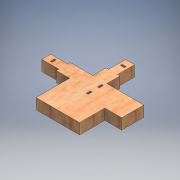
# Autodesk Inventor part: BearingStand_V2
Saved by Autodesk Inventor 2016 (Build 200138000, 138)
## iProperties
Created: 2015-11-23
Part Number: BearingStand_V2
Material: Wood (Birch)
Document SubType Name: Modeling
Designer: m2memari
Density: 0.55 g/cm^3
Appearance: Birch - Natural Polished
BearingDiameter: 24.000 mm
WoodThickness: 6.390 mm
BearingWidth: 7.000 mm
BearingShaftDiameter: 8.000 mm
ZipTieWidth: 2.500 mm
ZipTieThickness: 1.100 mm
ZipTieClearance: 1.000 mm
ZipTieDistance: 10.000 mm
BearingHolderHeight: 24.526 mm
BearingSiliconeWidth: 14.000 mm
Author: m2memari
Autodesk Inventor part; units mm, degrees
ref_plane "YZ Plane" through (0, 0, 0) normal (1, 0, 0) x (0, 1, 0)
ref_plane "XZ Plane" through (0, 0, 0) normal (0, 1, 0) x (-1, 0, 0)
ref_plane "XY Plane" through (0, 0, 0) normal (0, 0, 1) x (1, 0, 0)
sketch "Sketch1" plane through (0, 0, 0) normal (0, 0, 1) x (1, 0, 0)
  line L0 (-2.6473, 22.1) -> (2.6473, 22.1)
  line L1 (2.6473, 22.1) -> (2.6473, 12)
  line L2 (2.6473, 12) -> (4.1473, 12)
  line L3 (4.1473, 12) -> (4.1473, 4.1473)
  line L4 (0, 22.1) -> (0, 0) construction
  line L5 (-2.6473, 22.1) -> (-2.6473, 12)
  line L6 (-2.6473, 12) -> (-4.1473, 12)
  line L7 (-1.25, 18.6) -> (1.25, 18.6)
  line L8 (1.25, 18.6) -> (1.25, 17.5)
  line L9 (1.25, 17.5) -> (-1.25, 17.5)
  line L10 (-1.25, 17.5) -> (-1.25, 18.6)
  line L11 (-9.6473, -24) -> (16.1473, -24)
  line L12 (26.1473, -9) -> (16.1473, -9)
  line L13 (16.1473, -9) -> (16.1473, -24)
  line L14 (3.0473, 2.1473) -> (4.1473, 2.1473)
  line L15 (4.1473, 2.1473) -> (4.1473, -0.3527)
  line L16 (4.1473, -0.3527) -> (3.0473, -0.3527)
  line L17 (3.0473, -0.3527) -> (3.0473, 2.1473)
  line L18 (-4.1473, 12) -> (-30.8527, 12) construction
  line L19 (-27.6, 2.6473) -> (-27.6, -2.6473)
  line L20 (-27.6, -2.6473) -> (-17.5, -2.6473)
  line L21 (-17.5, -2.6473) -> (-17.5, -4.1473)
  line L22 (-17.5, -4.1473) -> (-9.6473, -4.1473)
  line L23 (-9.6473, -4.1473) -> (-9.6473, -24)
  line L24 (-27.6, 2.6473) -> (-17.5, 2.6473)
  line L25 (-17.5, 2.6473) -> (-17.5, 4.1473)
  line L26 (-24.1, 1.25) -> (-24.1, -1.25)
  line L27 (-24.1, -1.25) -> (-23, -1.25)
  line L28 (-23, -1.25) -> (-23, 1.25)
  line L29 (-23, 1.25) -> (-24.1, 1.25)
  line L30 (-17.5, 12) -> (-17.5, -24) construction
  line L31 (-4.1473, 12) -> (-4.1473, 4.1473)
  line L32 (-9.6473, 4.1473) -> (-17.5, 4.1473)
  line L33 (-4.1473, 4.1473) -> (-9.6473, 4.1473)
  line L34 (26.1473, 4.1473) -> (26.1473, -9)
  line L35 (26.1473, -2.4263) -> (4.1473, -2.4263) construction
  line L36 (3.0473, -7) -> (4.1473, -7)
  line L37 (4.1473, -7) -> (4.1473, -4.5)
  line L38 (4.1473, -4.5) -> (3.0473, -4.5)
  line L39 (3.0473, -4.5) -> (3.0473, -7)
  line L40 (4.1473, 4.1473) -> (26.1473, 4.1473)
  point P0 (0, 17.5)
  point P1 (3.0473, 0.8973)
  point P2 (4.1473, 0.8973)
  point P3 (-24.1, 0)
  point P4 (-27.6, 0)
  dimension "d4" = 1.5
  dimension "d26" = 10.1
  dimension "d27" = 5.2946
  dimension "d31" = 2.5
  dimension "d32" = 1.1
  dimension "d35" = 5.5
  dimension "d41" = 1.1
  dimension "d42" = 2.5
  dimension "d72" = 17.5
  dimension "BearingHolderHeight" = 24.5263
  dimension "d99" = 5.5
  dimension "d103" = 12
  dimension "d104" = 10
  dimension "d105" = 13.1473
  dimension "d106" = 2
  dimension "d108" = 15
  dimension "d124" = 12
  constraints: 82 end point, 23 perpendicular, 8 midpoint, 7 horizontal, 7 symmetric about line, 5 parallel, 4 horizontal alignment, 4 vertical alignment, 3 vertical, 2 collinear
  measures "d4" distance of L1.end L2.end
  measures "d26" distance of L0.end L1.end
  measures "d27" distance of L0.start L0.end
  measures "d31" distance of L7.start L7.end
  measures "d32" distance of L7.end L8.end
  measures "d35" distance between parallel lines of L6 L9
  measures "d41" distance of L15.end L16.end
  measures "d42" distance of L14.end L15.end
  measures "d72" distance between parallel lines of L30 L4
  measures "BearingHolderHeight" distance between parallel lines of L35 L0
  measures "d99" distance between parallel lines of L30 L28
  measures "d103" distance between parallel lines of L13 L3
  measures "d104" distance of L12.start L12.end
  measures "d105" distance of L34.start L12.start
  measures "d106" distance from line of L14.start L40
  measures "d108" distance of L12.end L11.end
  measures "d124" distance from line of point (-27.6, 0) L18
extrude "Extrusion2" add sketch "Sketch1" along normal blind 6.39
equation "\"BearingDiameter\" = 24"
equation "\"WoodThickness\" = 6.39"
equation "\"BearingWidth\" = 7"
equation "\"BearingShaftDiameter\" = 8"
equation "\"ZipTieWidth\" = 2.5"
equation "\"ZipTieThickness\" = 1.1"
equation "\"ZipTieClearance\" = 1"
equation "\"ZipTieDistance\" = 10"
equation "\"BearingSiliconeWidth\" = 14"
body "Solid2"
